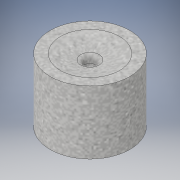
# Autodesk Inventor part: graphite
Saved by Autodesk Inventor 2017 (Build 210142000, 142)
## iProperties
Created: 2016-10-19
Part Number: graphite
Material: GFRC
Document SubType Name: Modeling
Designer: cflannery
Density: 1.7 g/cm^3
Appearance: Flat - Polished Gray
Author: cflannery
Autodesk Inventor part; units mm, degrees
ref_plane "YZ Plane" through (0, 0, 0) normal (1, 0, 0) x (0, 1, 0)
ref_plane "XZ Plane" through (0, 0, 0) normal (0, 1, 0) x (-1, 0, 0)
ref_plane "XY Plane" through (0, 0, 0) normal (0, 0, 1) x (1, 0, 0)
sketch "Sketch1" plane through (0, 0, 0) normal (0, 0, 1) x (1, 0, 0)
  line L0 (-24.002, 6.35) -> (-17.7813, 6.35)
  line L1 (-43.052, 13.1213) -> (-5.5282, 3.0668)
  line L2 (-3.4725, -1.3418) -> (-39.877, -79.4117)
  line L3 (-17.652, -31.75) -> (-24.002, -31.75)
  line L4 (-24.002, -31.75) -> (-24.002, 6.35)
  arc A0 (-3.4725, -1.3418) -> (-5.5282, 3.0668) centre (-6.35, 0) ccw
  line L5 (-30.352, 0.4213) -> (-30.352, -52.1764)
  line L6 (-30.352, -52.1764) -> (-27.177, -52.1764)
  line L7 (-30.352, 0.4213) -> (-43.052, 0.4213)
  line L8 (-43.052, 0.4213) -> (-43.052, 5.1238)
  line L9 (-43.052, 5.1238) -> (-43.052, 13.1213)
  line L10 (-43.052, 0.4213) -> (-43.052, -5.9287)
  line L11 (-43.052, -5.9287) -> (-36.702, -5.9287)
  line L12 (-36.702, -5.9287) -> (-36.702, -64.1466)
  line L13 (-36.702, -64.1466) -> (-32.7588, -64.1466)
  line L14 (-39.877, -5.9287) -> (-39.877, -9.1037)
  line L15 (-39.877, -9.1037) -> (-43.052, -9.1037)
  line L16 (-43.052, -9.1037) -> (-43.052, -21.8037)
  line L17 (-43.052, -21.8037) -> (-36.702, -21.8037)
  line L18 (-43.052, -51.4466) -> (-43.052, -79.4117)
  line L19 (-43.052, -51.4466) -> (-36.702, -51.4466)
  line L20 (-43.052, -79.4117) -> (-39.877, -79.4117)
  line L21 (0, -97.9183) -> (0, 31.6279) projected
  point P0 (0, 0)
  dimension "d0" = 6.35
  dimension "d1" = 25
  dimension "d2" = 15
  dimension "d4" = 6.35
  dimension "d5" = 38.1
  dimension "d6" = 31.75
  dimension "d7" = 6.35
  dimension "d11" = 6.35
  dimension "d13" = 12.7
  dimension "d15" = 6.35
  dimension "d16" = 6.35
  dimension "d18" = 3.175
  dimension "d19" = 12.7
  dimension "d20" = 3.175
  dimension "d21" = 6.35
  dimension "d22" = 3.175
  dimension "d23" = 3.175
  dimension "d24" = 6.35
  dimension "d25" = 12.7
  dimension "d26" = 58.2179
  dimension "d27" = 12.7
  constraints: 42 end point, 8 perpendicular, 6 point on line, 6 vertical, 5 horizontal, 2 point on circle, 2 tangent, 1 centre point, 1 horizontal alignment, 1 midpoint
  measures "d0" diameter of A0
  measures "d1" angle of L4 L2
  measures "d2" angle of L0 L1
  measures "d4" distance of point (0, 0) A0.centre
  measures "d5" distance of L3.end L0.start
  measures "d6" vertical distance of point (0, 0) L3.end
  measures "d7" distance between parallel lines of L4 L5
  measures "d11" distance of L3.start L3.end
  measures "d13" distance of L5.start L7.end
  measures "d15" distance between parallel lines of L5 L12
  measures "d16" distance between parallel lines of L7 L11
  measures "d18" distance of L5.end L6.end
  measures "d19" distance of L15.end L16.end
  measures "d20" distance of L14.end L15.end
  measures "d21" distance between parallel lines of L12 L16
  measures "d22" distance between parallel lines of L11 L15
  measures "d23" distance of L18.end L2.end
  measures "d24" distance of L18.start L19.end
  measures "d25" distance from line of L12.end L19
  measures "d26" distance of L11.end L12.end
  measures "d27" distance from line of L1.start L7
revolve "Revolution1" add sketch "Sketch1" angle 360 about axis through (0, -10, 0) along (0, 1, 0) contours L0 L1 A0 L2 L3 L4
body "Solid1"
